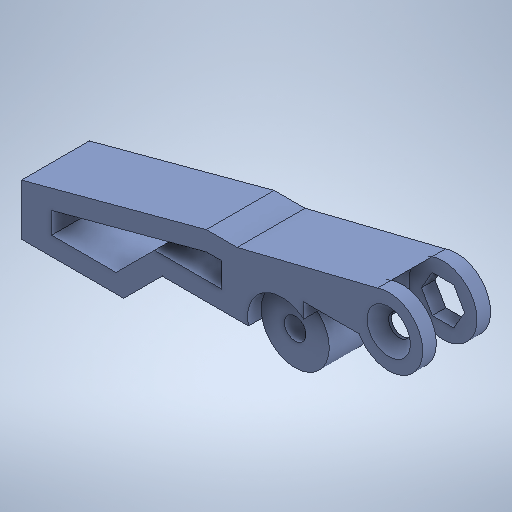
# Autodesk Inventor part: Pinza_0002_001
Saved by Autodesk Inventor 2025.2 (Build 292293000, 293)
## iProperties
Created: 2025-05-31
Part Number: Pinza_0002_001
Material: Borracha
Document SubType Name: Modeling
Designer: Gustavo Sousa
Density: 0.93 g/cm^3
Appearance: Borracha - Azul
Author: Gustavo Sousa
Autodesk Inventor part; units mm, degrees
ref_plane "YZ Plane" through (0, 0, 0) normal (1, 0, 0) x (0, 1, 0)
ref_plane "XZ Plane" through (0, 0, 0) normal (0, 1, 0) x (-1, 0, 0)
ref_plane "XY Plane" through (0, 0, 0) normal (0, 0, 1) x (1, 0, 0)
sketch "Esboço1" plane through (0, 0, 0) normal (0, 0, 1) x (1, 0, 0)
  circle A0 centre (28.2, 9.3) radius 5.5
  line L0 (-31.3, -7.5) -> (33.7, -7.5) construction
  line L1 (33.7, -7.5) -> (33.7, 14.8) construction
  line L2 (33.7, 14.8) -> (-31.3, 14.8) construction
  line L3 (-31.3, 14.8) -> (-31.3, -7.5) construction
  circle A1 centre (10.85, -0.05) radius 5.5
  line L4 (-14.7338, -7.5) -> (-8.5113, -1.2775)
  line L5 (-31.3, -7.5) -> (-14.7338, -7.5)
  line L6 (-8.5113, -1.2775) -> (5.4887, -1.2775)
  line L7 (-31.3, -7.5) -> (-31.3, 0.8)
  line L8 (-31.3, 0.8) -> (-1.3563, 8.8234)
  line L9 (-1.3563, 8.8234) -> (3.6437, 8.8234)
  line L10 (3.6437, 8.8234) -> (26.4006, 14.4973)
  line L11 (14.415, 4.1381) -> (14.415, 6.5881)
  line L12 (14.415, 6.5881) -> (23.415, 6.5881)
  line L13 (-26.4266, -1) -> (-26.4266, -4.5)
  line L14 (-26.4266, -4.5) -> (-15.9765, -4.5)
  line L15 (-26.4266, -1) -> (-1.3377, 5.7225)
  line L16 (-15.9765, -4.5) -> (-9.7539, 1.7225)
  line L17 (-9.7539, 1.7225) -> (1.1623, 1.7225)
  line L18 (1.1623, 1.7225) -> (1.1623, 5.7225)
  line L19 (1.1623, 5.7225) -> (-1.3377, 5.7225)
  point P0 (0, 0)
  dimension "d4" = 11
  dimension "d5" = 28.2
  dimension "d6" = 9.3
  dimension "d7" = 65
  dimension "d8" = 22.3
  dimension "d9" = 65
  dimension "d10" = 9.35
  dimension "d11" = 17.35
  dimension "d12" = 8.8
  dimension "d14" = 135
  dimension "d15" = 14
  dimension "d16" = 8.3
  dimension "d17" = 31
  dimension "d18" = 105
  dimension "d19" = 5
  dimension "d20" = 14
  dimension "d21" = 2.45
  dimension "d22" = 9
  dimension "d23" = 3
  dimension "d24" = 3
  dimension "d25" = 3.5
  dimension "d26" = 3
  dimension "d27" = 3
  dimension "d28" = 4
  dimension "d29" = 2.5
  constraints: 40 end point, 6 horizontal, 4 point on circle, 3 parallel, 3 vertical, 2 centre point, 2 point on line, 2 tangent, 1 collinear, 1 equal radius, 1 horizontal alignment, 1 perpendicular
  measures "d4" diameter of A0
  measures "d5" horizontal distance of A0.centre point (0, 0)
  measures "d6" vertical distance of point (0, 0) A0.centre
  measures "d7" distance of L1.end L2.end
  measures "d8" distance between parallel lines of L0 L2
  measures "d9" distance between parallel lines of L3 L1
  measures "d10" vertical distance of A0.centre A1.centre
  measures "d11" horizontal distance of A0.centre A1.centre
  measures "d12" distance of L4.start L4.end
  measures "d14" angle of L6 L4
  measures "d15" distance of L4.end L6.end
  measures "d16" distance of L0.start L7.end
  measures "d17" distance of L7.end L8.end
  measures "d18" angle of L8 L7
  measures "d19" distance of L8.end L9.end
  measures "d20" angle of L2 L10
  measures "d21" distance of L11.start L11.end
  measures "d22" distance of L11.end L12.end
  measures "d23" distance between parallel lines of L0 L14
  measures "d24" distance between parallel lines of L8 L15
  measures "d25" distance of L13.start L13.end
  measures "d26" distance between parallel lines of L4 L16
  measures "d27" distance between parallel lines of L6 L17
  measures "d28" distance of L17.end L18.end
  measures "d29" distance of L18.end L15.end
extrude "Extrusão1" add sketch "Esboço1" along normal blind 2.2 contours A0 L12 L11 A1 L6 L4 L5 L7 L8 L9 L10
extrude "Extrusão2" add sketch "Esboço1" against normal blind 6.6 contours A1
extrude "Extrusão3" add sketch "Esboço1" along normal blind 2.2 contours A0
sketch "Esboço2" plane through (0, 0, 0) normal (0, 0, 1) x (1, 0, 0)
  arc A0 (5.4887, -1.2775) -> (14.415, 4.1381) centre (10.85, -0.05) ccw projected
  point P0 (0, 0)
  constraints: 1 coincident
hole "Furo1" at (10.85, -0.05, 0) direction (0, 0, -1) diameter 3.5 end through all
sketch "Esboço3" plane through (0, 0, 2.2) normal (0, 0, 1) x (1, 0, 0)
  arc A0 (23.415, 6.5881) -> (26.4006, 14.4973) centre (28.2, 9.3) ccw projected
  point P0 (0, 0)
  constraints: 1 coincident
hole "Furo2" at (28.2, 9.3, 2.2) direction (0, 0, -1) diameter 3.5 end through all countersink diameter 7 countersink angle 90
pattern_linear "Padrão retangular3" count 2 spacing 8.8 along (0, 0, -1) of "Extrusão1", "Extrusão3"
sketch "Esboço6" plane through (-14.7338, -7.5, -8.8) normal (0, 0, -1) x (-1, 0, 0)
  circle A0 centre (-42.9338, 16.8) radius 3.5 projected
  line L0 (-41.1838, 13.7689) -> (-44.6838, 13.7689)
  line L1 (-44.6838, 13.7689) -> (-46.4338, 16.8)
  line L2 (-46.4338, 16.8) -> (-44.6838, 19.8311)
  line L3 (-44.6838, 19.8311) -> (-41.1838, 19.8311)
  line L4 (-41.1838, 19.8311) -> (-39.4338, 16.8)
  line L5 (-39.4338, 16.8) -> (-41.1838, 13.7689)
  point P0 (-14.7338, 7.5)
  point P1 (-42.9338, 16.8)
  constraints: 12 end point, 1 coincident, 1 horizontal alignment, 15 other
extrude "Extrusão6" cut sketch "Esboço6" along normal mid plane 4.4 contours L5 L0 L1 L2 L3 L4
sketch "Esboço4" plane through (0, 0, 0) normal (0, 0, -1) x (-1, 0, 0)
  line L0 (-26.4006, 14.4973) -> (-3.6437, 8.8234) projected
  line L1 (-26.4006, 14.4973) -> (-3.6437, 8.8234)
  line L2 (1.3563, 8.8234) -> (31.3, 0.8) projected
  line L3 (-3.6437, 8.8234) -> (1.3563, 8.8234)
  line L4 (1.3563, 8.8234) -> (31.3, 0.8)
  line L5 (31.3, 0.8) -> (31.3, -7.5)
  line L6 (31.3, -7.5) -> (14.7338, -7.5) projected
  line L7 (31.3, -7.5) -> (14.7338, -7.5)
  line L8 (14.7338, -7.5) -> (8.5113, -1.2775)
  line L9 (15.9765, -4.5) -> (9.7539, 1.7225) projected
  line L10 (8.5113, -1.2775) -> (-5.4887, -1.2775)
  arc A0 (-5.4887, -1.2775) -> (-14.415, 4.1381) centre (-10.85, -0.05) ccw projected
  arc A1 (-14.415, 4.1381) -> (-5.4887, -1.2775) centre (-10.85, -0.05) ccw
  line L11 (-14.415, 4.1381) -> (-14.415, 6.5881) projected
  line L12 (-14.415, 4.1381) -> (-14.415, 6.5881)
  line L13 (-14.415, 6.5881) -> (-23.415, 6.5881)
  line L14 (-14.415, 6.5881) -> (-23.415, 6.5881) projected
  arc A2 (-26.4006, 14.4973) -> (-23.415, 6.5881) centre (-28.2, 9.3) ccw construction
  arc A3 (-26.4006, 14.4973) -> (-23.415, 6.5881) centre (-28.2, 9.3) ccw projected
  arc A4 (-23.415, 6.5881) -> (-26.4006, 14.4973) centre (-28.2, 9.3) ccw
  line L15 (-1.1623, 5.7225) -> (1.3377, 5.7225) projected
  line L16 (-1.1623, 5.7225) -> (1.3377, 5.7225)
  line L17 (26.4266, -1) -> (1.3377, 5.7225) projected
  line L18 (1.3377, 5.7225) -> (26.4266, -1)
  line L19 (26.4266, -1) -> (26.4266, -4.5)
  line L20 (15.9765, -4.5) -> (26.4266, -4.5) projected
  line L21 (26.4266, -4.5) -> (15.9765, -4.5)
  line L22 (15.9765, -4.5) -> (9.7539, 1.7225)
  line L23 (9.7539, 1.7225) -> (-1.1623, 1.7225)
  line L24 (-1.1623, 1.7225) -> (-1.1623, 5.7225)
  point P0 (0, 0)
  point P1 (-5.4887, -1.2775)
  constraints: 32 end point, 6 point on circle, 5 collinear, 5 perpendicular, 3 centre point, 3 coincident, 3 horizontal, 2 parallel, 1 concentric
extrude "Extrusão7" add sketch "Esboço4" along normal blind 6.6 contours L0 L3 L2 L5 L6 L8 L10 A0 L11 L13 A4
